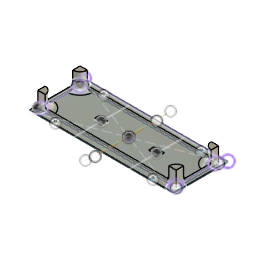
Stemmett Case Backplate (Autodesk Fusion 360 design; units mm, degrees)
Autodesk Fusion 360 part; units mm, degrees
sketch "Sketch1" plane through (0, 0, 0) normal (0, 0, 1) x (1, 0, 0)
  line L0 (107, 40.5) -> (-107, 40.5)
  line L1 (-107, 40.5) -> (-107, -40.5)
  line L2 (-107, -40.5) -> (107, -40.5)
  line L3 (107, -40.5) -> (107, 40.5)
  line L4 (107, 40.5) -> (-107, -40.5) construction
  line L5 (-107, 40.5) -> (107, -40.5) construction
  line L6 (-41.2, 40.5) -> (-41.2, -40.5)
  line L7 (41.2, 40.5) -> (41.2, -40.5)
  line L8 (-34.7, 2.75) -> (-47.7, 2.75)
  line L9 (-47.7, 2.75) -> (-47.7, -2.75)
  line L10 (-47.7, -2.75) -> (-34.7, -2.75)
  line L11 (-34.7, -2.75) -> (-34.7, 2.75)
  line L12 (-34.7, 2.75) -> (-47.7, -2.75) construction
  line L13 (-47.7, 2.75) -> (-34.7, -2.75) construction
  line L14 (46.35, 1.55) -> (36.05, 1.55)
  line L15 (36.05, 1.55) -> (36.05, -1.55)
  line L16 (36.05, -1.55) -> (46.35, -1.55)
  line L17 (46.35, -1.55) -> (46.35, 1.55)
  line L18 (46.35, 1.55) -> (36.05, -1.55) construction
  line L19 (36.05, 1.55) -> (46.35, -1.55) construction
  circle A0 centre (-72.6667, 35.5) radius 1.5
  line L20 (-0.1532, 41.6972) -> (-0.1532, -49.8073) construction
  line L21 (-0.1532, 41.6972) -> (-0.1532, -49.8073) construction
  circle A1 centre (72.3603, 35.5) radius 1.5
  circle A2 centre (-72.6667, -36.5) radius 1.5
  circle A3 centre (72.3603, -36.5) radius 1.5
  point P0 (-41.2, 0)
  point P1 (41.2, 0)
  dimension "d7" = 214
  dimension "d8" = 81
  dimension "d32" = 41.2
  dimension "d33" = 41.2
  dimension "d34" = 13
  dimension "d35" = 5.5
  dimension "d36" = 10.3
  dimension "d39" = 3.1
  dimension "d50" = 3
  dimension "d51" = 5
  dimension "d52" = 34.3333
  dimension "d55" = 3
  dimension "d56" = 4
  dimension "d57" = 34.3333
  constraint horizontal L0
  constraint perpendicular L0 L1
  constraint parallel L0 L2
  constraint parallel L1 L3
  constraint coincident L4 origin
  constraint coincident L5 origin
  constraint coincident L0 L6.start
  constraint coincident L2 L6.end
  constraint perpendicular L2 L6
  constraint coincident L0 L7.start
  constraint coincident L2 L7.end
  constraint perpendicular L2 L7
  constraint horizontal L8
  constraint perpendicular L8 L9
  constraint parallel L8 L10
  constraint parallel L9 L11
  constraint coincident L12 P0
  constraint coincident L13 P0
  constraint midpoint L6 P0
  constraint horizontal L14
  constraint perpendicular L14 L15
  constraint parallel L14 L16
  constraint parallel L15 L17
  constraint coincident L18 P1
  constraint coincident L19 P1
  constraint midpoint L7 P1
  constraint perpendicular L2 L20
  constraint symmetric A0 L20 A1
  constraint symmetric L21.start L20 L20.start
  constraint symmetric L21.end L20 L20.end
  constraint symmetric L21 A2 A3
  measures "d7" distance of L1 L3
  measures "d8" distance of L0 L2
  measures "d32" distance of origin L6
  measures "d33" distance of origin L7
  measures "d34" distance of L9 L11
  measures "d35" distance of L8 L10
  measures "d36" distance of L15 L17
  measures "d39" distance of L14 L16
  measures "d50" diameter of A0
  measures "d51" distance of L0 A0.centre
  measures "d52" distance of L1 A0.centre
  measures "d55" diameter of A2
  measures "d56" distance of L2 A2.centre
  measures "d57" distance of L1 A2.centre
extrude "Extrude1" add sketch "Sketch1" along normal blind 2.5 contours L0 L2 L3 L7 L14 L16 L17 | L0 L2 L6 L7 L8 L10 L11 L14 L15 L16 | L0 L1 L2 L6 L8 L9 L10 | L7 L14 L16 L17 | L7 L14 L15 L16 | L6 L8 L10 L11 | L6 L8 L9 L10 | A0 | A1 | A2 | A3
sketch "Sketch3" plane through (0, 0, 2.5) normal (0, 0, 1) x (-1, 0, 0)
  line L0 (-107, 40.5) -> (-107, -40.5)
  line L1 (-107, -40.5) -> (107, -40.5)
  line L2 (107, -40.5) -> (107, 40.5)
  line L3 (107, 40.5) -> (-107, 40.5)
  line L4 (103, -30.5) -> (-103, -30.5)
  line L5 (-103, -30.5) -> (-103, 32.5)
  line L6 (-103, 32.5) -> (103, 32.5)
  line L7 (103, 32.5) -> (103, -30.5)
  circle A0 centre (103, -30.5) radius 11
  circle A1 centre (103, 32.5) radius 11
  line L8 (0, -62.1045) -> (0, 64.593) construction
  circle A2 centre (-103, -30.5) radius 11
  circle A3 centre (-103, 32.5) radius 11
  line L9 (-100, -27.5) -> (-100, 29.5)
  line L10 (-100, 29.5) -> (100, 29.5)
  line L11 (100, 29.5) -> (100, -27.5)
  line L12 (100, -27.5) -> (-100, -27.5)
  line L13 (-107, -40.5) -> (107, -40.5)
  dimension "d14" = 8
  dimension "d15" = 206
  dimension "d16" = 63
  dimension "d17" = 4
  dimension "d18" = 4
  dimension "d20" = 22
  dimension "d21" = 22
  dimension "d26" = 3
  dimension "d59" = 10
  constraint horizontal L4
  constraint vertical L5
  constraint horizontal L6
  constraint vertical L7
  constraint coincident L4.start L7.end
  constraint coincident L6.end L7.start
  constraint vertical L8
  constraint symmetric A0 L8 A2
  constraint symmetric A1 L8 A3
  measures "d14" distance of L3 L6
  measures "d15" distance of L5 L7
  measures "d16" distance of L4 L6
  measures "d17" distance of L2 L7
  measures "d18" distance of L0 L5
  measures "d20" diameter of A0
  measures "d21" diameter of A1
  measures "d59" distance of L4 L13
extrude "Extrude2" add sketch "Sketch3" along normal blind 23 contours L5 L6 A3 L9 L10 | L4 L5 A2 L9 L12 | A3 L9 L10 | L6 L7 A1 L10 L11 | A2 L9 L12 | A1 L10 L11 | L4 L7 A0 L11 L12 | A0 L11 L12
extrude "Extrude3" add sketch "Sketch3" along normal blind 3 contours L5 A2 A3 L9 | L6 A1 A3 L10 | L4 A0 A2 L12 | L7 A0 A1 L11
sketch "Sketch4" plane through (0, 0, 2.5) normal (0, 0, 1) x (-1, 0, 0)
  line L0 (100, 29.5) -> (100, -27.5)
  line L1 (-100, -27.5) -> (-100, 29.5)
  dimension "d29" = 200
  measures "d29" distance of L0 L1
extrude "Extrude4" cut sketch "Sketch1" along normal blind 2.5 contours L7 L14 L16 L17 | L7 L14 L15 L16 | L6 L8 L10 L11 | L6 L8 L9 L10
chamfer "Chamfer1" distance 1 angle 45 4 edges at (0, 40.5, 0) (107, 0, 0) (0, -40.5, 0) (-107, 0, 0)
fillet "Fillet1" radius 10 12 edges at (-95.2218, 22.7218, 2.5) (92.417, 27.5, 4) (95.2218, 22.7218, 2.5) (-92.417, 27.5, 4) (-100, 19.917, 4) (-100, -21.917, 4) (100, -21.917, 4) (95.2218, -24.7218, 2.5) (100, 19.917, 4) (92.417, -29.5, 4) (-95.2218, -24.7218, 2.5) (-92.417, -29.5, 4)
sketch "Sketch5" plane through (0, 0, 0) normal (0, 0, 1) x (1, 0, 0)
  line L0 (-40.4637, -7.2967) -> (41.9799, -7.2967) construction
  line L1 (41.9799, -7.2967) -> (41.9799, -28.9026) construction
  line L2 (41.9799, -28.9026) -> (-40.4637, -28.9026) construction
  line L3 (-40.4637, -28.9026) -> (-40.4637, -7.2967) construction
  dimension "d45" = 11
chamfer "Chamfer2" distance 2.5 angle 45 4 edges at (41.2, -1.55, 2.5) (46.35, 0, 2.5) (41.2, 1.55, 2.5) (36.05, 0, 2.5)
extrude "Extrude6" cut sketch "Sketch1" along normal up to surface (2.5 mm away) contours A0 | A1 | A2 | A3
equation "CaseInnerWidth = 206 mm"
equation "CaseInnerHeight = 63 mm"
equation "CaseLipTopH = 10 mm"
equation "CaseLipW = 4 mm"
equation "SupportPillarHeight = 23 mm"
equation "d7 = CaseLipW + CaseInnerWidth + CaseLipW"
equation "d8 = CaseLipTopH + CaseInnerHeight + CaseLipBottomH"
equation "CaseLipThickness = 2.5 mm"
equation "d10 = CaseLipThickness"
equation "d14 = CaseLipBottomH"
equation "d15 = CaseInnerWidth"
equation "d16 = CaseInnerHeight"
equation "d17 = CaseLipW"
equation "SupperPillarRadius = 11 mm"
equation "d20 = SupperPillarRadius * 2"
equation "d21 = 2 * SupperPillarRadius"
equation "d22 = SupportPillarHeight"
equation "CaseInnerLipThickness = 3 mm"
equation "CaseInnerLipWidth = 3 mm"
equation "d26 = CaseInnerLipWidth"
equation "d27 = CaseInnerLipThickness"
equation "UsbJackH = 5.5 mm"
equation "UsbJackW = 13 mm"
equation "d32 = CaseInnerWidth / 5"
equation "d33 = CaseInnerWidth / 5"
equation "d34 = UsbJackW"
equation "d35 = UsbJackH"
equation "d36 = LightSensorW"
equation "LightSensorW = 10.3 mm"
equation "LightSensorH = 3.1 mm"
equation "d39 = LightSensorH"
equation "d40 = CaseLipThickness"
equation "d46 = 'STEMMETT'"
equation "d51 = CaseLipTopH / 2"
equation "d52 = CaseInnerWidth / 6"
equation "d56 = CaseLipBottomH / 2"
equation "d57 = CaseInnerWidth / 6"
equation "CaseLipBottomH = 8 mm"
